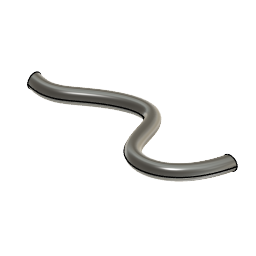
Sweep Command Hollow Pipe (Autodesk Fusion 360 design; units mm, degrees)
part number: 2026-06-14-15-47-05-341
Autodesk Fusion 360 part; units mm, degrees
sketch "Sketch1" plane through (0, 0, 0) normal (0, 0, 1) x (1, 0, 0)
  spline S0 degree 5 poles (0, 0) (2.3965, -0.7913) (7.1096, -2.1712) (13.9395, -3.6328) (22.5657, -4.3629) (32.6026, -3.2525) (42.065, -0.1661) (51.3077, 4.785) (60.9182, 11.3986) (71.5341, 19.3535) (83.6707, 28.1784) (97.5533, 37.2255) (112.923, 45.6288) (128.9181, 52.3013) (144.3944, 56.1454) (158.1835, 56.2343) (169.3842, 52.013) (177.6209, 43.4779) (183.3737, 31.4129) (187.7236, 17.1669) (192.0184, 2.3697) (197.5569, -11.337) (205.2932, -22.5526) (215.46, -30.4332) (227.6702, -34.6402) (241.1806, -35.1652) (255.0916, -32.2031) (268.5879, -25.9994) (281.1131, -16.7357) (292.3015, -4.549) (301.944, 10.4672) (308.3429, 24.6966) (312.3906, 36.6024) (314.7557, 45.0868) (315.8549, 49.4658) knots 0 0 0 0 0 0 0.033333 0.066667 0.1 0.133333 0.166667 0.2 0.233333 0.266667 0.3 0.333333 0.366667 0.4 0.433333 0.466667 0.5 0.533333 0.566667 0.6 0.633333 0.666667 0.7 0.733333 0.766667 0.8 0.833333 0.866667 0.9 0.933333 0.966667 1 1 1 1 1 1
  point P0 (41.2971, 0)
  point P1 (95.5279, 35.6244)
  point P2 (170, 50)
  point P3 (199.9053, -13.8413)
  point P4 (252.3208, -32.2208)
  constraint coincident S0.start origin
sketch "Sketch2" plane through (0, 0, 0) normal (1, 0, 0) x (0, 1, 0)
  circle A0 centre (0, 0) radius 12.5
  circle A1 centre (0, 0) radius 11.5
  dimension "d1" = 25
  dimension "d2" = 23
  constraint coincident A0.centre A1.centre
  constraint concentric A0 A1
  measures "d1" diameter of A0
  measures "d2" diameter of A1
sweep "Sweep1" add profiles "Sketch2" path "Sketch1" along S0 section 1
